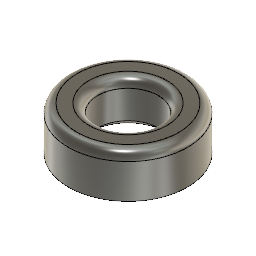
SpacerM5x4 (Autodesk Fusion 360 design; units mm, degrees)
Autodesk Fusion 360 part; units mm, degrees
sketch "Sketch1" plane through (0, 0, 0) normal (0, 0, 1) x (1, 0, 0)
  circle A0 centre (0, 0) radius 2.8
  circle A1 centre (0, 0) radius 5.5
  dimension "d1" = 5.6
  dimension "d2" = 2.7
  constraint coincident A0.centre A1.centre
  measures "d1" diameter of A0
extrude "Extrude1" add sketch "Sketch1" along normal blind 4
chamfer "Chamfer1" distance 0.6 angle 45 1 edges at (-2.6105, 1.0125, 0)
fillet "Fillet1" radius 0.8 1 faces at (4.5691, -0.4124, 4)
